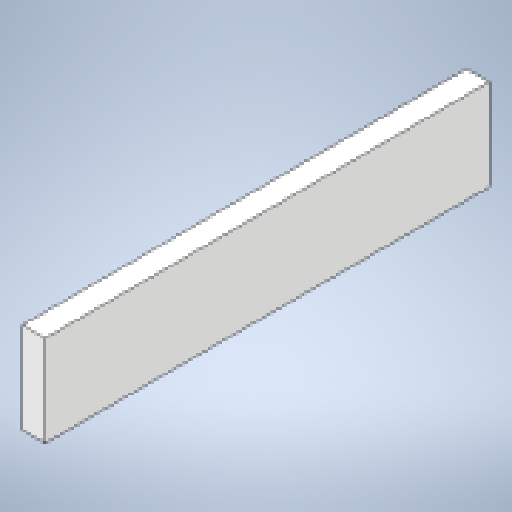
# Autodesk Inventor part: Back_Plate
Saved by Autodesk Inventor 2023.2 (Build 272271000, 271)
## iProperties
Created: 2024-01-26
Part Number: Back_Plate
Material: UHMW, White
Document SubType Name: Modeling
Designer: Nathan Cai
Mass: 19.2548 g
Surface Area: 83.8708 cm^2
Volume: 20.4838 cm^3
Density: 0.94 g/cm^3
Appearance: Smooth - White
Author: Nathan Cai
Autodesk Inventor part; units mm, degrees
ref_plane "YZ Plane" through (0, 0, 0) normal (1, 0, 0) x (0, 1, 0)
ref_plane "XZ Plane" through (0, 0, 0) normal (0, 1, 0) x (-1, 0, 0)
ref_plane "XY Plane" through (0, 0, 0) normal (0, 0, 1) x (1, 0, 0)
sketch "Sketch1" plane through (0, 0, 0) normal (1, 0, 0) x (0, 1, 0)
  line L0 (-12.7, 61.9125) -> (12.7, 61.9125)
  line L1 (12.7, 61.9125) -> (12.7, -61.9125)
  line L2 (12.7, -61.9125) -> (-12.7, -61.9125)
  line L3 (-12.7, -61.9125) -> (-12.7, 61.9125)
  line L4 (-12.7, 61.9125) -> (12.7, -61.9125) construction
  line L5 (12.7, 61.9125) -> (-12.7, -61.9125) construction
  point P0 (0, 0)
  dimension "d0" = 25.4
  dimension "d1" = 123.825
  constraints: 12 end point, 2 midpoint, 2 parallel, 1 horizontal, 1 perpendicular
  measures "d0" distance of L1.end L2.end
  measures "d1" distance of L0.end L1.end
extrude "Extrusion1" add sketch "Sketch1" along normal blind 6.35
body "Solid1"
